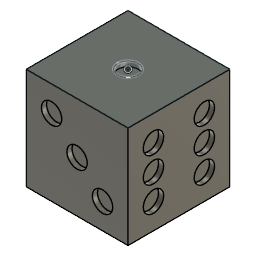
Die (Autodesk Fusion 360 design; units mm, degrees)
part number: 2026-07-19-19-57-33-454
Autodesk Fusion 360 part; units mm, degrees
sketch "Sketch1" plane through (0, 0, 0) normal (0, 0, 1) x (1, 0, 0)
  line L0 (10, -10) -> (-10, -10)
  line L1 (-10, -10) -> (-10, 10)
  line L2 (-10, 10) -> (10, 10)
  line L3 (10, 10) -> (10, -10)
  line L4 (10, -10) -> (-10, 10) construction
  line L5 (-10, -10) -> (10, 10) construction
  dimension "d1" = 20
  dimension "d2" = 20
  constraint horizontal L0
  constraint perpendicular L0 L1
  constraint parallel L0 L2
  constraint parallel L1 L3
  constraint coincident L4 origin
  constraint coincident L5 origin
  measures "d1" distance of L1.end L2.end
  measures "d2" distance of L0.end L1.end
extrude "Extrude1" add sketch "Sketch1" along normal mid plane 20
sketch "Sketch2" plane through (0, 0, 10) normal (0, 0, 1) x (-1, 0, 0)
  line L0 (-10, -10) -> (10, -10)
  line L1 (10, -10) -> (10, 10)
  line L2 (10, 10) -> (-10, 10)
  line L3 (-10, 10) -> (-10, -10)
  circle A0 centre (0, 0) radius 2
  dimension "d5" = 4
  constraint coincident A0.centre origin
  measures "d5" diameter of A0
extrude "Extrude2" cut sketch "Sketch2" against normal blind 1 contours A0
sketch "Sketch3" plane through (0, -10, 0) normal (0, -1, 0) x (1, 0, 0)
  line L0 (10, -10) -> (10, 10)
  line L1 (10, 10) -> (-10, 10)
  line L2 (-10, 10) -> (-10, -10)
  line L3 (-10, -10) -> (10, -10)
  line L4 (-10, 10) -> (10, -10) construction
  circle A0 centre (0, 0) radius 2
  circle A1 centre (-5, 5) radius 2
  circle A2 centre (5, -5) radius 2
  dimension "d8" = 4
  dimension "d9" = 4
  dimension "d10" = 4
  constraint coincident L1.end L2.start
  constraint coincident L0.start L3.end
  constraint coincident A0.centre origin
  constraint coincident L4 A1.centre
  constraint coincident L4 A2.centre
  measures "d8" diameter of A0
  measures "d9" diameter of A1
  measures "d10" diameter of A2
extrude "Extrude3" cut sketch "Sketch3" against normal blind 1 contours A0 | A1 | A2
sketch "Sketch4" plane through (-10, 0, 0) normal (-1, 0, 0) x (0, -1, 0)
  line L0 (10, -10) -> (10, 10)
  line L1 (10, 10) -> (-10, 10)
  line L2 (-10, 10) -> (-10, -10)
  line L3 (-10, -10) -> (10, -10)
  line L4 (-10, 10) -> (10, -10) construction
  line L5 (10, 10) -> (-10, -10) construction
  circle A0 centre (0, 0) radius 2
  circle A1 centre (-5, 5) radius 2
  circle A2 centre (5, 5) radius 2
  circle A3 centre (-5, -5) radius 2
  circle A4 centre (5, -5) radius 2
  dimension "d13" = 4
  dimension "d14" = 4
  dimension "d15" = 4
  dimension "d16" = 4
  constraint coincident L1.end L2.start
  constraint coincident L0.start L3.end
  constraint coincident L0.end L1.start
  constraint coincident L2.end L3.start
  constraint coincident A0.centre origin
  constraint coincident L4 A1.centre
  constraint coincident L5 A2.centre
  constraint coincident L5 A3.centre
  constraint coincident L4 A4.centre
  constraint equal A0 A4
  measures "d13" diameter of A0
  measures "d14" diameter of A1
  measures "d15" diameter of A2
  measures "d16" diameter of A3
extrude "Extrude4" cut sketch "Sketch4" against normal blind 1 contours A0 | A1 | A2 | A3 | A4
sketch "Sketch5" plane through (0, 10, 0) normal (0, 1, 0) x (-1, 0, 0)
  line L0 (10, -10) -> (10, 10)
  line L1 (10, 10) -> (-10, 10)
  line L2 (-10, 10) -> (-10, -10)
  line L3 (-10, -10) -> (10, -10)
  line L4 (-10, 10) -> (10, -10) construction
  circle A0 centre (-5, 5) radius 2
  circle A1 centre (5, -5) radius 2
  dimension "d19" = 4
  dimension "d20" = 4
  constraint coincident L1.end L2.start
  constraint coincident L0.start L3.end
  constraint coincident L4 A0.centre
  constraint coincident L4 A1.centre
  measures "d19" diameter of A0
  measures "d20" diameter of A1
extrude "Extrude5" cut sketch "Sketch5" against normal blind 1 contours A0 | A1
sketch "Sketch6" plane through (10, 0, 0) normal (1, 0, 0) x (0, 1, 0)
  line L0 (10, -10) -> (10, 10)
  line L1 (10, 10) -> (-10, 10)
  line L2 (-10, 10) -> (-10, -10)
  line L3 (-10, -10) -> (10, -10)
  line L4 (-10, 10) -> (10, -10) construction
  line L5 (10, 10) -> (-10, -10) construction
  line L6 (-10, 0) -> (10, 0) construction
  line L7 (0, 10) -> (0, -10) construction
  circle A0 centre (-5, 0) radius 2
  circle A1 centre (-5, 5) radius 2
  circle A2 centre (-5, -5) radius 2
  circle A3 centre (5, 5) radius 2
  circle A4 centre (5, 0) radius 2
  circle A5 centre (5, -5) radius 2
  dimension "d23" = 4
  dimension "d24" = 4
  dimension "d25" = 4
  dimension "d26" = 4
  dimension "d27" = 4
  dimension "d28" = 4
  constraint coincident L1.end L2.start
  constraint coincident L0.start L3.end
  constraint coincident L0.end L1.start
  constraint coincident L2.end L3.start
  constraint midpoint L2 L6.start
  constraint midpoint L0 L6.end
  constraint midpoint L1 L7.start
  constraint midpoint L3 L7.end
  constraint coincident L6 A0.centre
  constraint coincident L4 A1.centre
  constraint coincident L5 A2.centre
  constraint coincident L5 A3.centre
  constraint coincident L6 A4.centre
  constraint coincident L4 A5.centre
  measures "d23" diameter of A0
  measures "d24" diameter of A1
  measures "d25" diameter of A2
  measures "d26" diameter of A3
  measures "d27" diameter of A4
  measures "d28" diameter of A5
extrude "Extrude6" cut sketch "Sketch6" against normal blind 1 contours A0 | A1 | A2 | A3 | A4 | A5
sketch "Sketch7" plane through (0, 0, -10) normal (0, 0, -1) x (1, 0, 0)
  line L0 (-10, -10) -> (10, -10)
  line L1 (10, -10) -> (10, 10)
  line L2 (10, 10) -> (-10, 10)
  line L3 (-10, 10) -> (-10, -10)
  line L4 (10, 10) -> (-10, -10) construction
  line L5 (10, -10) -> (-10, 10) construction
  circle A0 centre (5, 5) radius 2
  circle A1 centre (-5, -5) radius 2
  circle A2 centre (-5, 5) radius 2
  circle A3 centre (5, -5) radius 2
  dimension "d31" = 4
  dimension "d32" = 4
  dimension "d33" = 4
  constraint coincident L1.end L2.start
  constraint coincident L0.start L3.end
  constraint coincident L0.end L1.start
  constraint coincident L2.end L3.start
  constraint coincident L4 A0.centre
  constraint coincident L4 A1.centre
  constraint coincident L5 A2.centre
  constraint coincident L5 A3.centre
  constraint equal A1 A3
  measures "d31" diameter of A0
  measures "d32" diameter of A1
  measures "d33" diameter of A2
extrude "Extrude7" cut sketch "Sketch7" against normal blind 1 contours A0 | A1 | A2 | A3
equation "d1 = diceSize"
equation "d2 = diceSize"
equation "d3 = diceSize"
equation "diceSize = 20 mm"
equation "DivotDia = 4 mm"
